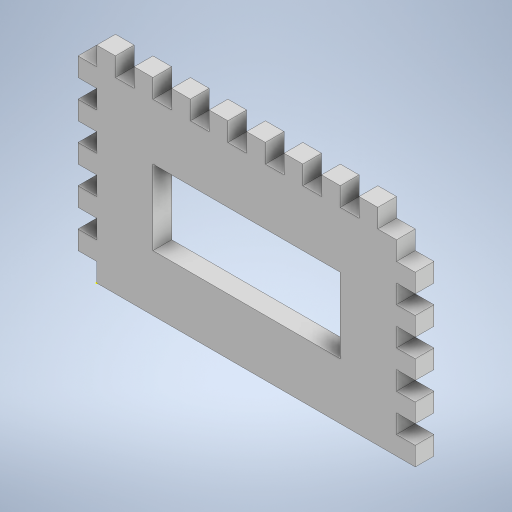
# Autodesk Inventor part: leftrightsidehole
Saved by Autodesk Inventor 2024 (Build 280153000, 153)
## iProperties
Created: 2024-04-15
Part Number: leftrightsidehole
Material: Generic
Document SubType Name: Modeling
Designer: srika
Density: 1 g/cm^3
Appearance: Default
Author: srika
Autodesk Inventor part; units mm, degrees
ref_plane "YZ Plane" through (0, 0, 0) normal (1, 0, 0) x (0, 1, 0)
ref_plane "XZ Plane" through (0, 0, 0) normal (0, 1, 0) x (-1, 0, 0)
ref_plane "XY Plane" through (0, 0, 0) normal (0, 0, 1) x (1, 0, 0)
sketch "Sketch1" plane through (0, 0, 0) normal (0, 0, 1) x (1, 0, 0)
  line L0 (0, 0) -> (5, 0)
  line L1 (5, 0) -> (5, 5)
  line L2 (5, 5) -> (0, 5)
  line L3 (0, 5) -> (0, 0)
  line L4 (5, 5) -> (85, 5)
  line L5 (85, 5) -> (85, 55)
  line L6 (85, 55) -> (5, 55)
  line L7 (5, 55) -> (5, 5)
  line L8 (0, 10) -> (5, 10)
  line L9 (5, 10) -> (5, 15)
  line L10 (5, 15) -> (0, 15)
  line L11 (0, 15) -> (0, 10)
  line L12 (0, 20) -> (5, 20)
  line L13 (5, 20) -> (5, 25)
  line L14 (5, 25) -> (0, 25)
  line L15 (0, 25) -> (0, 20)
  line L16 (0, 30) -> (5, 30)
  line L17 (5, 30) -> (5, 35)
  line L18 (5, 35) -> (0, 35)
  line L19 (0, 35) -> (0, 30)
  line L20 (0, 40) -> (5, 40)
  line L21 (5, 40) -> (5, 45)
  line L22 (5, 45) -> (0, 45)
  line L23 (0, 45) -> (0, 40)
  line L24 (0, 50) -> (5, 50)
  line L25 (5, 50) -> (5, 55)
  line L26 (5, 55) -> (0, 55)
  line L27 (0, 55) -> (0, 50)
  line L28 (10, 0) -> (15, 0)
  line L29 (15, 0) -> (15, 5)
  line L30 (15, 5) -> (10, 5)
  line L31 (10, 5) -> (10, 0)
  line L32 (20, 0) -> (25, 0)
  line L33 (25, 0) -> (25, 5)
  line L34 (25, 5) -> (20, 5)
  line L35 (20, 5) -> (20, 0)
  line L36 (30, 0) -> (35, 0)
  line L37 (35, 0) -> (35, 5)
  line L38 (35, 5) -> (30, 5)
  line L39 (30, 5) -> (30, 0)
  line L40 (40, 0) -> (45, 0)
  line L41 (45, 0) -> (45, 5)
  line L42 (45, 5) -> (40, 5)
  line L43 (40, 5) -> (40, 0)
  line L44 (50, 0) -> (55, 0)
  line L45 (55, 0) -> (55, 5)
  line L46 (55, 5) -> (50, 5)
  line L47 (50, 5) -> (50, 0)
  line L48 (60, 0) -> (65, 0)
  line L49 (65, 0) -> (65, 5)
  line L50 (65, 5) -> (60, 5)
  line L51 (60, 5) -> (60, 0)
  line L52 (70, 0) -> (75, 0)
  line L53 (75, 0) -> (75, 5)
  line L54 (75, 5) -> (70, 5)
  line L55 (70, 5) -> (70, 0)
  line L56 (80, 0) -> (85, 0)
  line L57 (85, 0) -> (85, 5)
  line L58 (85, 5) -> (80, 5)
  line L59 (80, 5) -> (80, 0)
  line L60 (85, 55) -> (90, 55)
  line L61 (90, 55) -> (90, 60)
  line L62 (90, 60) -> (85, 60)
  line L63 (85, 60) -> (85, 55)
  line L64 (75, 55) -> (80, 55)
  line L65 (75, 60) -> (75, 55)
  line L66 (80, 55) -> (80, 60)
  line L67 (80, 60) -> (75, 60)
  line L68 (65, 55) -> (70, 55)
  line L69 (65, 60) -> (65, 55)
  line L70 (70, 55) -> (70, 60)
  line L71 (70, 60) -> (65, 60)
  line L72 (55, 55) -> (60, 55)
  line L73 (55, 60) -> (55, 55)
  line L74 (60, 55) -> (60, 60)
  line L75 (60, 60) -> (55, 60)
  line L76 (45, 55) -> (50, 55)
  line L77 (45, 60) -> (45, 55)
  line L78 (50, 55) -> (50, 60)
  line L79 (50, 60) -> (45, 60)
  line L80 (35, 55) -> (40, 55)
  line L81 (35, 60) -> (35, 55)
  line L82 (40, 55) -> (40, 60)
  line L83 (40, 60) -> (35, 60)
  line L84 (25, 55) -> (30, 55)
  line L85 (25, 60) -> (25, 55)
  line L86 (30, 55) -> (30, 60)
  line L87 (30, 60) -> (25, 60)
  line L88 (15, 55) -> (20, 55)
  line L89 (15, 60) -> (15, 55)
  line L90 (20, 55) -> (20, 60)
  line L91 (20, 60) -> (15, 60)
  line L92 (5, 55) -> (10, 55)
  line L93 (5, 60) -> (5, 55)
  line L94 (10, 55) -> (10, 60)
  line L95 (10, 60) -> (5, 60)
  line L96 (85, 45) -> (90, 45)
  line L97 (90, 45) -> (90, 50)
  line L98 (90, 50) -> (85, 50)
  line L99 (85, 50) -> (85, 45)
  line L100 (85, 35) -> (90, 35)
  line L101 (90, 35) -> (90, 40)
  line L102 (90, 40) -> (85, 40)
  line L103 (85, 40) -> (85, 35)
  line L104 (85, 25) -> (90, 25)
  line L105 (90, 25) -> (90, 30)
  line L106 (90, 30) -> (85, 30)
  line L107 (85, 30) -> (85, 25)
  line L108 (85, 15) -> (90, 15)
  line L109 (90, 15) -> (90, 20)
  line L110 (90, 20) -> (85, 20)
  line L111 (85, 20) -> (85, 15)
  line L112 (85, 5) -> (90, 5)
  line L113 (90, 5) -> (90, 10)
  line L114 (90, 10) -> (85, 10)
  line L115 (85, 10) -> (85, 5)
  dimension "d0" = 5
  dimension "d1" = 5
  dimension "d2" = 80
  dimension "d3" = 50
  dimension "d6" = 10
  dimension "d13" = 10
  dimension "d18" = 5
  dimension "d19" = 5
  dimension "d22" = 10
  dimension "d29" = 10
  constraints: 232 end point, 6 parallel, 5 horizontal, 3 perpendicular, 2 vertical, 208 other
  measures "d0" distance of L2.end L1.end
  measures "d1" distance of L1.end L0.end
  measures "d2" distance of L6.end L5.end
  measures "d3" distance of L5.end L4.end
  measures "d6" distance of L0.start L8.start
  measures "d13" distance of L0.start L28.start
  measures "d18" distance of L62.end L61.end
  measures "d19" distance of L61.end L60.end
  measures "d22" distance of L5.end L64.start
  measures "d29" distance of L5.end L96.start
sketch "Sketch2" plane through (0, 0, 0) normal (0, 0, 1) x (1, 0, 0)
  point P0 (0, 0)
sketch "Sketch3" plane through (0, 0, 0) normal (0, 0, 1) x (1, 0, 0)
  line L0 (20, 20) -> (70, 20)
  line L1 (70, 20) -> (70, 40)
  line L2 (70, 40) -> (20, 40)
  line L3 (20, 40) -> (20, 20)
  point P0 (0, 0)
  dimension "d34" = 50
  dimension "d35" = 20
  constraints: 8 end point, 2 parallel, 1 horizontal, 1 perpendicular
  measures "d34" distance of L2.end L1.end
  measures "d35" distance of L1.end L0.end
extrude "Extrusion1" add sketch "Sketch1" along normal blind 5 contours L7 L6 L5 L4 | L8 L11 L10 L7 | L12 L15 L14 L7 | L16 L19 L18 L7 | L20 L23 L22 L7 | L24 L27 L26 L7 | L93 L95 L94 L6 | L89 L91 L90 L6 | L85 L87 L86 L6 | L5 L114 L113 L112 | L81 L83 L82 L6 | L5 L110 L109 L108 | L77 L79 L78 L6 | L5 L106 L105 L104 | L73 L75 L74 L6 | L5 L102 L101 L100 | L69 L71 L70 L6 | L5 L98 L97 L96 | L65 L67 L66 L6
extrude "Extrusion2" cut sketch "Sketch3" along normal blind 10
body "Solid1"
